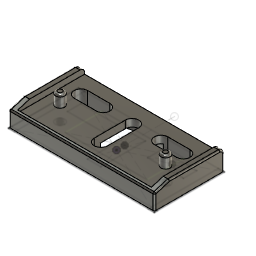
ATIthingie (Autodesk Fusion 360 design; units mm, degrees)
Autodesk Fusion 360 part; units mm, degrees
sketch "Sketch1" plane through (0, 0, 0) normal (0, 0, 1) x (1, 0, 0)
  line L0 (49, 23.5) -> (-49, 23.5)
  line L1 (-49, 23.5) -> (-49, -23.5)
  line L2 (-49, -23.5) -> (49, -23.5)
  line L3 (49, -23.5) -> (49, 23.5)
  line L4 (49, 23.5) -> (-49, -23.5) construction
  line L5 (-49, 23.5) -> (49, -23.5) construction
  line L6 (4.5, 15) -> (-4.5, 15)
  line L7 (-4.5, 15) -> (-4.5, -15)
  line L8 (-4.5, -15) -> (4.5, -15)
  line L9 (4.5, -15) -> (4.5, 15)
  line L10 (4.5, 15) -> (-4.5, -15) construction
  line L11 (-4.5, 15) -> (4.5, -15) construction
  line L12 (49, 23.5) -> (45, 23.5)
  line L13 (45, 23.5) -> (45, -23.5)
  line L14 (45, -23.5) -> (49, -23.5)
  line L15 (49, -23.5) -> (49, 23.5)
  line L16 (-49, 23.5) -> (-45, 23.5)
  line L17 (-45, 23.5) -> (-45, -23.5)
  line L18 (-45, -23.5) -> (-49, -23.5)
  line L19 (-49, -23.5) -> (-49, 23.5)
  line L20 (27.5, 18) -> (-27.5, 18)
  line L21 (-27.5, 18) -> (-27.5, -7)
  line L22 (-27.5, -7) -> (27.5, -7)
  line L23 (27.5, -7) -> (27.5, 18)
  line L24 (27.5, 18) -> (-27.5, -7) construction
  line L25 (-27.5, 18) -> (27.5, -7) construction
  line L26 (39, 15) -> (15, 15)
  line L27 (15, 15) -> (15, 6)
  line L28 (15, 6) -> (39, 6)
  line L29 (39, 6) -> (39, 15)
  line L30 (39, 15) -> (15, 6) construction
  line L31 (15, 15) -> (39, 6) construction
  line L32 (0, 0) -> (0, 39) construction
  line L33 (-39, 15) -> (-15, 15)
  line L34 (-39, 6) -> (-39, 15)
  line L35 (-15, 6) -> (-39, 6)
  line L36 (-15, 15) -> (-15, 6)
  line L37 (-49, -23.5) -> (49, -23.5)
  line L38 (49, -23.5) -> (49, -21.5)
  line L39 (49, -21.5) -> (-49, -21.5)
  line L40 (-49, -21.5) -> (-49, -23.5)
  circle A0 centre (35.5, -2.5) radius 3
  circle A1 centre (-35.5, -2.5) radius 3
  point P0 (0, 5.5)
  point P1 (0, 5.5)
  point P2 (27, 10.5)
  dimension "d1" = 98
  dimension "d2" = 47
  dimension "d3" = 9
  dimension "d4" = 30
  dimension "d5" = 4
  dimension "d6" = 47
  dimension "d7" = 4
  dimension "d8" = 47
  dimension "d13" = 18
  dimension "d14" = 55
  dimension "d15" = 25
  dimension "d34" = 24
  dimension "d35" = 9
  dimension "d36" = 13
  dimension "d38" = 22
  dimension "d69" = 98
  dimension "d70" = 2
  dimension "d73" = 6
  dimension "d74" = 21
  dimension "d75" = 13.5
  constraint horizontal L0
  constraint perpendicular L0 L1
  constraint parallel L0 L2
  constraint parallel L1 L3
  constraint coincident L4 L32.start
  constraint coincident L5 L32.start
  constraint coincident L32.start origin
  constraint horizontal L6
  constraint perpendicular L6 L7
  constraint parallel L6 L8
  constraint parallel L7 L9
  constraint coincident L10 L32.start
  constraint coincident L11 L32.start
  constraint horizontal L12
  constraint vertical L13
  constraint horizontal L14
  constraint vertical L15
  constraint horizontal L16
  constraint vertical L17
  constraint horizontal L18
  constraint vertical L19
  constraint horizontal L20
  constraint perpendicular L20 L21
  constraint parallel L20 L22
  constraint parallel L21 L23
  constraint coincident L24 P1
  constraint coincident L25 P1
  constraint coincident P1 P0
  constraint horizontal L26
  constraint perpendicular L26 L27
  constraint parallel L26 L28
  constraint parallel L27 L29
  constraint coincident L30 P2
  constraint coincident L31 P2
  constraint vertical L32
  constraint symmetric L26.start L32 L33.start
  constraint symmetric L26.end L32 L33.end
  constraint symmetric L27.end L32 L35.start
  constraint symmetric L28.end L32 L34.start
  constraint horizontal L37
  constraint vertical L38
  constraint horizontal L39
  constraint vertical L40
  constraint symmetric L32 A0 A1
  measures "d1" distance of L1.end L2.end
  measures "d2" distance of L0.end L1.end
  measures "d3" distance of L7.end L8.end
  measures "d4" distance of L6.end L7.end
  measures "d5" distance of L0.start L12.end
  measures "d6" distance of L0.start L2.end
  measures "d7" distance of L0.end L16.end
  measures "d8" distance of L0.end L1.end
  measures "d13" distance of L0 P1
  measures "d14" distance of L21.end L22.end
  measures "d15" distance of L20.end L21.end
  measures "d34" distance of L27.end L28.end
  measures "d35" distance of L26.end L27.end
  measures "d36" distance of L0 P2
  measures "d38" distance of L3 P2
  measures "d69" distance of L1.end L2.end
  measures "d70" distance of L1.end L39.end
  measures "d73" diameter of A0
  measures "d74" distance of L2 A0.centre
  measures "d75" distance of L3 A0.centre
extrude "Extrude4" add sketch "Sketch1" along normal blind 10 contours L0 L3 L12 L13 L15 L39 | L0 L13 L17 L39 | L2 L3 L13 L14 L15 L37 L38 L39 | L0 L1 L16 L17 L19 L39 | L2 L13 L17 L37 L39 | L1 L2 L17 L18 L19 L37 L39 L40 | L6 L7 L9 L22 | L6 L7 L9 L20 L21 L22 L23 L26 L27 L28 L33 L35 L36 | L7 L8 L9 L22 | L23 L26 L27 L28 | L23 L26 L28 L29 | L21 L33 L34 L35 | L21 L33 L35 L36 | A0 | A1 in component "Bracket body"
extrude "Extrude5" cut sketch "Sketch1" along normal blind 5 contours L6 L7 L9 L22 | L6 L7 L9 L20 L21 L22 L23 L26 L27 L28 L33 L35 L36 | L23 L26 L27 L28 | L21 L33 L35 L36 in component "Bracket body"
chamfer "Chamfer3" distance 26 distance2 6 1 edges at (27.5, 18, 2.5) measured on face at (9.1667, 18, 1.6667) in component "Bracket body"
chamfer "Chamfer3" distance 6 distance2 26 1 edges at (-27.5, 18, 2.5) measured on face at (-27.5, 9.6667, 1.6667) in component "Bracket body"
chamfer "Chamfer3" distance 26 distance2 6 1 edges at (-27.5, -7, 2.5) measured on face at (-9.1667, -7, 1.6667) in component "Bracket body"
chamfer "Chamfer3" distance 6 distance2 26 1 edges at (27.5, -7, 2.5) measured on face at (27.5, 1.3333, 1.6667) in component "Bracket body"
fillet "Fillet4" radius 8 4 edges at (27.5, 12, 2.5) (-27.5, 12, 2.5) (-27.5, -1, 2.5) (27.5, -1, 2.5) in component "Bracket body"
extrude "Extrude6" cut sketch "Sketch1" along normal blind 10 contours L6 L7 L9 L22 | L7 L8 L9 L22 | L23 L26 L27 L28 | L23 L26 L28 L29 | L21 L33 L34 L35 | L21 L33 L35 L36 in component "Bracket body"
extrude "Extrude7" add sketch "Sketch1" along normal blind 14 contours L0 L3 L12 L13 L15 L39 | L2 L3 L13 L14 L15 L37 L38 L39 | L0 L1 L16 L17 L19 L39 | L1 L2 L17 L18 L19 L37 L39 L40 in component "Bracket body"
extrude "Extrude8" add sketch "Sketch1" along normal blind 12 contours L2 L13 L17 L37 L39 in component "Bracket body"
chamfer "Chamfer4" distance 10 distance2 3 2 edges at (47, -23.5, 14) (-47, -23.5, 14) measured on face at (46.3333, -7.8333, 14) measured on face at (-47.6667, -7.8333, 14) in component "Bracket body"
fillet "Fillet7" radius 1 9 edges at (0, -23.5, 11) (49, 5, 14) (49, -23.5, 5.5) (49, -18.5, 12.5) (-49, -23.5, 5.5) (-49, 5, 14) (-49, -18.5, 12.5) (49, 23.5, 7) (-49, 23.5, 7) in component "Bracket body"
chamfer "Chamfer5" distance 0.5 angle 45 8 edges at (49, 0, 0) (48.7071, 23.2071, 0) (0, 23.5, 0) (-48.7071, 23.2071, 0) (-49, 0, 0) (-48.7071, -23.2071, 0) (0, -23.5, 0) (48.7071, -23.2071, 0) in component "Bracket body"
fillet "Fillet5" radius 3 2 edges at (47, 23.5, 14) (-47, 23.5, 14) in component "Bracket body"
fillet "Fillet6" radius 4.5 4 edges at (39, 15, 5) (15, 15, 5) (15, 6, 7.5) (39, 6, 5) in component "Bracket body"
fillet "Fillet6" radius 4.5 4 edges at (-39, 15, 5) (-39, 6, 5) (-15, 6, 7.5) (-15, 15, 5) in component "Bracket body"
fillet "Fillet6" radius 4.5 4 edges at (4.5, 15, 7.5) (-4.5, 15, 7.5) (-4.5, -15, 5) (4.5, -15, 5) in component "Bracket body"
extrude "Extrude10" cut sketch "Sketch1" along normal blind 10 contours A0 | A1 in component "Bracket body"
extrude "Extrude11" add sketch "Sketch1" along normal blind 13 from surface at 5 contours A0 | A1 in component "Bracket body"
fillet "Fillet8" radius 1.5 2 faces at (-35.7973, -0.5279, 18) (35.2027, -0.5279, 18) in component "Bracket body"
component "Bracket body" placed x (1, 0, 0) y (0, 1, 0) z (0, 0, 1) at (0, 0, 0)
